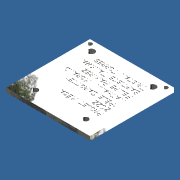
# Autodesk Inventor part: PlaqueGuideBlocLame
Saved by Autodesk Inventor 2018 (Build 220112000, 112)
## iProperties
Created: 2022-03-10
Part Number: PlaqueGuideBlocLame
Material: Aluminum 6061
Document SubType Name: Modeling
Designer: Nathann
Density: 2.7 g/cm^3
Appearance: Aluminum - Flat
Mass: 132.189 g
Surface Area: 221.993 cm^2
Volume: 48.9589 cm^3
Author: Nathann
Autodesk Inventor part; units mm, degrees
(part 1 of 3)
ref_plane "YZ Plane" through (0, 0, 0) normal (1, 0, 0) x (0, 1, 0)
ref_plane "XZ Plane" through (0, 0, 0) normal (0, 1, 0) x (-1, 0, 0)
ref_plane "XY Plane" through (0, 0, 0) normal (0, 0, 1) x (1, 0, 0)
sketch "Sketch1" plane through (0, 0, 0) normal (0, 0, 1) x (1, 0, 0)
  line L0 (0, 0) -> (-100, 0)
  line L1 (-100, 0) -> (-100, 100)
  line L2 (-100, 100) -> (0, 100)
  line L3 (0, 100) -> (0, 0)
  dimension "d0" = 100
  dimension "d1" = 100
  constraints: 8 end point, 2 parallel, 1 horizontal, 1 perpendicular
  measures "d0" distance of L2.end L0.start
  measures "d1" distance of L1.end L2.end
extrude "Extrusion1" add sketch "Sketch1" along normal blind 5
sketch "Sketch11" plane through (-80, 15, 0) normal (0, 0, -1) x (-1, 0, 0)
  circle A0 centre (0, 0) radius 3.3
  circle A1 centre (-30, 0) radius 5 projected
  circle A2 centre (-30, 0) radius 3
  circle A3 centre (-60, 0) radius 5 projected
  circle A4 centre (-60, 0) radius 3.3
  point P0 (-80, -15)
  dimension "d101" = 6.6
  dimension "d102" = 6
  dimension "d103" = 6.6
  constraints: 3 centre point, 2 coincident
  measures "d101" diameter of A0
  measures "d102" diameter of A2
  measures "d103" diameter of A4
extrude "Extrusion11" cut sketch "Sketch11" along normal through all both and the other way through all contours A0 | A4
sketch "Sketch7" plane through (0, 0, 0) normal (0, 0, -1) x (-1, 0, 0)
  line L0 (100, 25) -> (0, 25)
  line L1 (100, 56.2495) -> (100, 25)
  line L2 (100, 100) -> (0, 100)
  line L3 (0, 0) -> (100, 0) projected
  circle A0 centre (86.5, 88) radius 4
  circle A1 centre (86.5, 88) radius 1.65
  line L4 (50, 100) -> (50, 0)
  line L5 (100, 0) -> (0, 0) projected
  line L6 (0, 100) -> (0, 100)
  line L7 (0, 100) -> (0, 98.5)
  circle A2 centre (95, 95) radius 2.5
  line L8 (100, 0) -> (100, 100) projected
  line L9 (0, 0) -> (100, 0) projected
  line L10 (100, 0) -> (100, 100) projected
  line L11 (100, 100) -> (0, 100) projected
  line L12 (0, 100) -> (0, 0) projected
  circle A3 centre (13.5, 88) radius 4
  circle A4 centre (13.5, 88) radius 1.65
  circle A5 centre (5, 95) radius 2.5
  point P0 (95.4835, 97.4528)
  point P1 (95.4244, 97.4637)
  point P2 (0, 100)
  point P3 (0, 100)
  point P4 (4.5165, 97.4528)
  point P5 (4.5756, 97.4637)
  point P6 (0, 100)
  dimension "d72" = 25
  dimension "d77" = 8
  dimension "d78" = 3.3
  dimension "d88" = 5
  dimension "d111" = 5
  dimension "d112" = 8.5
  dimension "d121" = 7
  dimension "d122" = 5
  constraints: 12 end point, 8 symmetric about line, 6 centre point, 4 point on circle, 2 coincident, 2 horizontal, 2 midpoint, 3 other
  measures "d72" distance between parallel lines of L0 L3
  measures "d77" diameter of A0
  measures "d78" diameter of A1
  measures "d88" diameter of A2
  measures "d111" distance from line of L8 A2.centre
  measures "d112" horizontal distance of A2.centre A0.centre
  measures "d121" vertical distance of A0.centre A2.centre
  measures "d122" distance from line of L2 A2.centre
extrude "Extrusion13" cut sketch "Sketch7" against normal blind 10 contours A0 | A1 | A2 | A3 | A4 | A5
sketch "Sketch13" plane through (0, 0, 5) normal (0, 0, 1) x (1, 0, 0)
  line L0 (-10, 25) -> (-90, 25) construction
  line L1 (-90, 25) -> (-90, 85) construction
  line L2 (-90, 85) -> (-10, 85) construction
  line L3 (-10, 85) -> (-10, 25) construction
  line L4 (0, 0) -> (0, 100) projected
  line L5 (-100, 100) -> (-100, 0) projected
  line L6 (-100, 0) -> (0, 0) projected
  spline S0 degree 2 poles (-14.4043, 27.4336) (-14.4043, 28.1165) (-14.0606, 28.4281) knots 0 0 0 1 1 1
  spline S1 degree 2 poles (-14.0606, 28.4281) (-13.6527, 28.9735) (-12.9606, 28.9735) knots 0 0 0 1 1 1
  line L7 (-12.9606, 28.9735) -> (-11.1778, 28.9735)
  line L8 (-11.1778, 28.9735) -> (-11.1778, 31.5446)
  spline S2 degree 2 poles (-11.1778, 31.5446) (-11.1778, 31.9066) (-10.8295, 31.9066) knots 0 0 0 1 1 1
  spline S3 degree 2 poles (-10.8295, 31.9066) (-10.4766, 31.9066) (-10.4766, 31.5446) knots 0 0 0 1 1 1
  line L9 (-10.4766, 31.5446) -> (-10.4766, 25.8249)
  line L10 (-10.4766, 25.8249) -> (-12.8186, 25.8249)
  spline S4 degree 2 poles (-12.8186, 25.8249) (-13.6114, 25.8249) (-14.0285, 26.2832) knots 0 0 0 1 1 1
  spline S5 degree 2 poles (-14.0285, 26.2832) (-14.4043, 26.7095) (-14.4043, 27.4336) knots 0 0 0 1 1 1
  spline S6 degree 2 poles (-13.7031, 27.4336) (-13.7031, 26.5307) (-12.8186, 26.5307) knots 0 0 0 1 1 1
  line L11 (-12.8186, 26.5307) -> (-11.1778, 26.5307)
  line L12 (-11.1778, 26.5307) -> (-11.1778, 28.2585)
  line L13 (-11.1778, 28.2585) -> (-12.9652, 28.2585)
  spline S7 degree 2 poles (-12.9652, 28.2585) (-13.3181, 28.2585) (-13.7031, 27.814) (-13.7031, 27.4336) knots 0 0 0 1 2 2 2
  spline S8 degree 2 poles (-18.9415, 28.3089) (-18.9415, 29.0651) (-18.4694, 29.4134) knots 0 0 0 1 1 1
  spline S9 degree 2 poles (-18.4694, 29.4134) (-18.0936, 29.7205) (-17.7499, 29.7205) knots 0 0 0 1 1 1
  line L14 (-17.7499, 29.7205) -> (-17.7086, 29.7159)
  line L15 (-17.7086, 29.7159) -> (-18.8727, 31.3337)
  spline S10 degree 2 poles (-18.8727, 31.3337) (-18.9415, 31.4437) (-18.9415, 31.5446) knots 0 0 0 1 1 1
  spline S11 degree 2 poles (-18.9415, 31.5446) (-18.9415, 31.6912) (-18.7261, 31.9066) (-18.584, 31.9066) knots 0 0 0 1 2 2 2
  spline S12 degree 2 poles (-18.584, 31.9066) (-18.419, 31.9066) (-18.3778, 31.7966) knots 0 0 0 1 1 1
  line L16 (-18.3778, 31.7966) -> (-16.9295, 29.7205)
  line L17 (-16.9295, 29.7205) -> (-16.0817, 29.7205)
  line L18 (-16.0817, 29.7205) -> (-16.0817, 31.5446)
  spline S13 degree 2 poles (-16.0817, 31.5446) (-16.0817, 31.9066) (-15.7334, 31.9066) knots 0 0 0 1 1 1
  spline S14 degree 2 poles (-15.7334, 31.9066) (-15.385, 31.9066) (-15.385, 31.5446) knots 0 0 0 1 1 1
  line L19 (-15.385, 31.5446) -> (-15.385, 26.8928)
  line L20 (-15.385, 26.8928) -> (-17.4932, 26.8928)
  spline S15 degree 2 poles (-17.4932, 26.8928) (-18.0936, 26.8928) (-18.4969, 27.2503) knots 0 0 0 1 1 1
  spline S16 degree 2 poles (-18.4969, 27.2503) (-18.9415, 27.649) (-18.9415, 28.3089) knots 0 0 0 1 1 1
  spline S17 degree 2 poles (-18.2449, 28.3089) (-18.2449, 27.9652) (-17.8095, 27.5986) (-17.4932, 27.5986) knots 0 0 0 1 2 2 2
  line L21 (-17.4932, 27.5986) -> (-16.0817, 27.5986)
  line L22 (-16.0817, 27.5986) -> (-16.0817, 29.0147)
  line L23 (-16.0817, 29.0147) -> (-17.7499, 29.0147)
  spline S18 degree 2 poles (-17.7499, 29.0147) (-17.8782, 29.0147) (-18.0386, 28.8681) knots 0 0 0 1 1 1
  spline S19 degree 2 poles (-18.0386, 28.8681) (-18.2449, 28.6756) (-18.2449, 28.3089) knots 0 0 0 1 1 1
  spline S20 degree 2 poles (-23.3458, 29.3951) (-23.3458, 30.3667) (-22.8554, 31.0954) knots 0 0 0 1 1 1
  spline S21 degree 2 poles (-22.8554, 31.0954) (-22.3146, 31.8974) (-21.4667, 31.8974) knots 0 0 0 1 1 1
  spline S22 degree 2 poles (-21.4667, 31.8974) (-20.6189, 31.8974) (-20.0781, 31.0863) knots 0 0 0 1 1 1
  spline S23 degree 2 poles (-20.0781, 31.0863) (-19.5923, 30.3576) (-19.5923, 29.3951) knots 0 0 0 1 1 1
  spline S24 degree 2 poles (-19.5923, 29.3951) (-19.5923, 28.4373) (-20.0735, 27.7269) knots 0 0 0 1 1 1
  spline S25 degree 2 poles (-20.0735, 27.7269) (-20.6372, 26.9065) (-21.4667, 26.9065) knots 0 0 0 1 1 1
  spline S26 degree 2 poles (-21.4667, 26.9065) (-22.3512, 26.9065) (-22.8233, 27.6719) knots 0 0 0 1 1 1
  spline S27 degree 2 poles (-22.8233, 27.6719) (-23.3458, 28.4235) (-23.3458, 29.3951) knots 0 0 0 1 1 1
  spline S28 degree 2 poles (-22.6491, 29.3951) (-22.6491, 28.6802) (-22.3833, 28.2219) knots 0 0 0 1 1 1
  spline S29 degree 2 poles (-22.3833, 28.2219) (-22.0396, 27.6123) (-21.4667, 27.6123) knots 0 0 0 1 1 1
  spline S30 degree 2 poles (-21.4667, 27.6123) (-20.9305, 27.6123) (-20.5914, 28.1806) knots 0 0 0 1 1 1
  spline S31 degree 2 poles (-20.5914, 28.1806) (-20.2889, 28.6939) (-20.2889, 29.3951) knots 0 0 0 1 1 1
  spline S32 degree 2 poles (-20.2889, 29.3951) (-20.2889, 30.1147) (-20.4447, 30.5821) knots 0 0 0 1 1 1
  spline S33 degree 2 poles (-20.4447, 30.5821) (-20.9122, 31.1917) (-21.4667, 31.1917) knots 0 0 0 1 1 1
  spline S34 degree 2 poles (-21.4667, 31.1917) (-22.0258, 31.1917) (-22.4933, 30.5821) knots 0 0 0 1 1 1
  spline S35 degree 2 poles (-22.4933, 30.5821) (-22.6491, 30.1101) (-22.6491, 29.3951) knots 0 0 0 1 1 1
  spline S36 degree 2 poles (-27.2597, 30.1788) (-27.2597, 30.8113) (-26.8105, 31.2696) knots 0 0 0 1 1 1
  spline S37 degree 2 poles (-26.8105, 31.2696) (-26.2835, 31.9158) (-25.5227, 31.9158) knots 0 0 0 1 1 1
  spline S38 degree 2 poles (-25.5227, 31.9158) (-24.8857, 31.9158) (-24.3953, 31.3887) knots 0 0 0 1 1 1
  spline S39 degree 2 poles (-24.3953, 31.3887) (-23.9324, 30.8892) (-23.9324, 30.3484) knots 0 0 0 1 1 1
  spline S40 degree 2 poles (-23.9324, 30.3484) (-23.9324, 29.9955) (-24.2715, 29.9955) knots 0 0 0 1 1 1
  spline S41 degree 2 poles (-24.2715, 29.9955) (-24.629, 29.9955) (-24.629, 30.3667) knots 0 0 0 1 1 1
  spline S42 degree 2 poles (-24.629, 30.3667) (-24.629, 30.6554) (-25.1744, 31.2192) (-25.5273, 31.2192) knots 0 0 0 1 2 2 2
  spline S43 degree 2 poles (-25.5273, 31.2192) (-25.9764, 31.2192) (-26.2606, 30.9213) knots 0 0 0 1 1 1
  spline S44 degree 2 poles (-26.2606, 30.9213) (-26.563, 30.5592) (-26.563, 30.1788) knots 0 0 0 1 1 1
  line L24 (-26.563, 30.1788) -> (-26.563, 27.2457)
  spline S45 degree 2 poles (-26.563, 27.2457) (-26.563, 26.8836) (-26.9113, 26.8836) knots 0 0 0 1 1 1
  spline S46 degree 2 poles (-26.9113, 26.8836) (-27.2597, 26.8836) (-27.2597, 27.2457) knots 0 0 0 1 1 1
  line L25 (-27.2597, 27.2457) -> (-27.2597, 30.1788)
  line L26 (-31.224, 31.8287) -> (-28.2404, 31.8287)
  line L27 (-28.2404, 31.8287) -> (-28.2404, 26.8928)
  line L28 (-28.2404, 26.8928) -> (-31.224, 26.8928)
  spline S47 degree 2 poles (-31.224, 26.8928) (-31.5814, 26.8928) (-31.5814, 27.2365) knots 0 0 0 1 1 1
  spline S48 degree 2 poles (-31.5814, 27.2365) (-31.5814, 27.5894) (-31.224, 27.5894) knots 0 0 0 1 1 1
  line L29 (-31.224, 27.5894) -> (-28.937, 27.5894)
  line L30 (-28.937, 27.5894) -> (-28.937, 28.7489)
  line L31 (-28.937, 28.7489) -> (-31.0865, 28.7489)
  spline S49 degree 2 poles (-31.0865, 28.7489) (-31.4348, 28.7489) (-31.4348, 29.1018) knots 0 0 0 1 1 1
  spline S50 degree 2 poles (-31.4348, 29.1018) (-31.4348, 29.4547) (-31.0865, 29.4547) knots 0 0 0 1 1 1
  line L32 (-31.0865, 29.4547) -> (-28.937, 29.4547)
  line L33 (-28.937, 29.4547) -> (-28.937, 31.1229)
  line L34 (-28.937, 31.1229) -> (-31.224, 31.1229)
  spline S51 degree 2 poles (-31.224, 31.1229) (-31.5814, 31.1229) (-31.5814, 31.4758) knots 0 0 0 1 1 1
  spline S52 degree 2 poles (-31.5814, 31.4758) (-31.5814, 31.8287) (-31.224, 31.8287) knots 0 0 0 1 1 1
  line L35 (-35.8803, 27.6169) -> (-34.6979, 27.6169)
  line L36 (-34.6979, 27.6169) -> (-34.6979, 31.5446)
  spline S53 degree 2 poles (-34.6979, 31.5446) (-34.6979, 31.9158) (-34.3404, 31.9158) knots 0 0 0 1 1 1
  spline S54 degree 2 poles (-34.3404, 31.9158) (-33.9784, 31.9158) (-33.9784, 31.5446) knots 0 0 0 1 1 1
  line L37 (-33.9784, 31.5446) -> (-33.9784, 27.6169)
  line L38 (-33.9784, 27.6169) -> (-32.8005, 27.6169)
  spline S55 degree 2 poles (-32.8005, 27.6169) (-32.4385, 27.6169) (-32.4385, 27.2548) knots 0 0 0 1 1 1
  spline S56 degree 2 poles (-32.4385, 27.2548) (-32.4385, 26.8928) (-32.8005, 26.8928) knots 0 0 0 1 1 1
  line L39 (-32.8005, 26.8928) -> (-35.8803, 26.8928)
  spline S57 degree 2 poles (-35.8803, 26.8928) (-36.247, 26.8928) (-36.247, 27.2548) knots 0 0 0 1 1 1
  spline S58 degree 2 poles (-36.247, 27.2548) (-36.247, 27.6169) (-35.8803, 27.6169) knots 0 0 0 1 1 1
  spline S59 degree 2 poles (-45.3992, 31.5446) (-45.3992, 31.9066) (-45.0509, 31.9066) knots 0 0 0 1 1 1
  spline S60 degree 2 poles (-45.0509, 31.9066) (-44.698, 31.9066) (-44.698, 31.5446) knots 0 0 0 1 1 1
  line L40 (-44.698, 31.5446) -> (-44.698, 26.9386)
  line L41 (-44.698, 26.9386) -> (-43.3094, 29.1339)
  spline S61 degree 2 poles (-43.3094, 29.1339) (-43.149, 29.3676) (-42.9198, 29.3676) knots 0 0 0 1 1 1
  spline S62 degree 2 poles (-42.9198, 29.3676) (-42.6999, 29.3676) (-42.5853, 29.198) knots 0 0 0 1 1 1
  line L42 (-42.5853, 29.198) -> (-41.1691, 26.9203)
  line L43 (-41.1691, 26.9203) -> (-41.1691, 31.5446)
  spline S63 degree 2 poles (-41.1691, 31.5446) (-41.1691, 31.9066) (-40.8116, 31.9066) knots 0 0 0 1 1 1
  spline S64 degree 2 poles (-40.8116, 31.9066) (-40.4588, 31.9066) (-40.4588, 31.5446) knots 0 0 0 1 1 1
  line L44 (-40.4588, 31.5446) -> (-40.4588, 26.2237)
  spline S65 degree 2 poles (-40.4588, 26.2237) (-40.4588, 25.8433) (-40.8391, 25.8433) knots 0 0 0 1 1 1
  spline S66 degree 2 poles (-40.8391, 25.8433) (-41.1325, 25.8433) (-41.3249, 26.1137) knots 0 0 0 1 1 1
  line L45 (-41.3249, 26.1137) -> (-42.929, 28.4831)
  line L46 (-42.929, 28.4831) -> (-44.5697, 26.0862)
  spline S67 degree 2 poles (-44.5697, 26.0862) (-44.7576, 25.8066) (-45.0234, 25.8066) knots 0 0 0 1 1 1
  spline S68 degree 2 poles (-45.0234, 25.8066) (-45.3992, 25.8066) (-45.3992, 26.2191) knots 0 0 0 1 1 1
  line L47 (-45.3992, 26.2191) -> (-45.3992, 31.5446)
  line L48 (-49.744, 31.8287) -> (-46.7604, 31.8287)
  line L49 (-46.7604, 31.8287) -> (-46.7604, 26.8928)
  line L50 (-46.7604, 26.8928) -> (-49.744, 26.8928)
  spline S69 degree 2 poles (-49.744, 26.8928) (-50.1014, 26.8928) (-50.1014, 27.2365) knots 0 0 0 1 1 1
  spline S70 degree 2 poles (-50.1014, 27.2365) (-50.1014, 27.5894) (-49.744, 27.5894) knots 0 0 0 1 1 1
  line L51 (-49.744, 27.5894) -> (-47.457, 27.5894)
  line L52 (-47.457, 27.5894) -> (-47.457, 28.7489)
  line L53 (-47.457, 28.7489) -> (-49.6065, 28.7489)
  spline S71 degree 2 poles (-49.6065, 28.7489) (-49.9548, 28.7489) (-49.9548, 29.1018) knots 0 0 0 1 1 1
  spline S72 degree 2 poles (-49.9548, 29.1018) (-49.9548, 29.4547) (-49.6065, 29.4547) knots 0 0 0 1 1 1
  line L54 (-49.6065, 29.4547) -> (-47.457, 29.4547)
  line L55 (-47.457, 29.4547) -> (-47.457, 31.1229)
  line L56 (-47.457, 31.1229) -> (-49.744, 31.1229)
  spline S73 degree 2 poles (-49.744, 31.1229) (-50.1014, 31.1229) (-50.1014, 31.4758) knots 0 0 0 1 1 1
  spline S74 degree 2 poles (-50.1014, 31.4758) (-50.1014, 31.8287) (-49.744, 31.8287) knots 0 0 0 1 1 1
  line L57 (-49.5286, 25.6462) -> (-48.3782, 26.2557)
  spline S75 degree 2 poles (-48.3782, 26.2557) (-48.2866, 26.3016) (-48.2041, 26.3016) knots 0 0 0 1 1 1
  spline S76 degree 2 poles (-48.2041, 26.3016) (-48.062, 26.3016) (-47.8695, 26.0724) (-47.8695, 25.9395) knots 0 0 0 1 2 2 2
  spline S77 degree 2 poles (-47.8695, 25.9395) (-47.8695, 25.7608) (-48.0528, 25.6554) knots 0 0 0 1 1 1
  line L58 (-48.0528, 25.6554) -> (-49.194, 25.0367)
  spline S78 degree 2 poles (-49.194, 25.0367) (-49.2673, 25) (-49.3498, 25) knots 0 0 0 1 1 1
  spline S79 degree 2 poles (-49.3498, 25) (-49.4965, 25) (-49.689, 25.2292) (-49.689, 25.3712) knots 0 0 0 1 2 2 2
  spline S80 degree 2 poles (-49.689, 25.3712) (-49.689, 25.55) (-49.5286, 25.6462) knots 0 0 0 1 1 1
  spline S81 degree 2 poles (-54.5011, 31.0954) (-54.107, 31.5721) (-53.4104, 31.9158) (-52.92, 31.9158) knots 0 0 0 1 2 2 2
  spline S82 degree 2 poles (-52.92, 31.9158) (-52.1271, 31.9158) (-51.1143, 30.5088) (-51.1143, 29.3539) knots 0 0 0 1 2 2 2
  spline S83 degree 2 poles (-51.1143, 29.3539) (-51.1143, 28.0798) (-51.7192, 27.4198) knots 0 0 0 1 1 1
  spline S84 degree 2 poles (-51.7192, 27.4198) (-52.2096, 26.8836) (-52.92, 26.8836) knots 0 0 0 1 1 1
  spline S85 degree 2 poles (-52.92, 26.8836) (-53.4516, 26.8836) (-54.1253, 27.2594) (-54.3911, 27.7406) knots 0 0 0 1 2 2 2
  spline S86 degree 2 poles (-54.3911, 27.7406) (-54.4324, 27.8186) (-54.4324, 27.9056) knots 0 0 0 1 1 1
  spline S87 degree 2 poles (-54.4324, 27.9056) (-54.4324, 28.0477) (-54.2124, 28.2539) (-54.0749, 28.2539) knots 0 0 0 1 2 2 2
  spline S88 degree 2 poles (-54.0749, 28.2539) (-53.8824, 28.2539) (-53.7816, 28.0706) knots 0 0 0 1 1 1
  spline S89 degree 2 poles (-53.7816, 28.0706) (-53.5112, 27.5894) (-52.9383, 27.5894) knots 0 0 0 1 1 1
  spline S90 degree 2 poles (-52.9383, 27.5894) (-52.4983, 27.5894) (-52.205, 27.9515) knots 0 0 0 1 1 1
  spline S91 degree 2 poles (-52.205, 27.9515) (-51.8155, 28.4418) (-51.8155, 29.3539) knots 0 0 0 1 1 1
  spline S92 degree 2 poles (-51.8155, 29.3539) (-51.8155, 30.1926) (-52.4708, 31.2192) (-52.9383, 31.2192) knots 0 0 0 1 2 2 2
  spline S93 degree 2 poles (-52.9383, 31.2192) (-53.5204, 31.2192) (-53.9099, 30.8021) knots 0 0 0 1 1 1
  spline S94 degree 2 poles (-53.9099, 30.8021) (-54.0382, 30.5363) (-54.2032, 30.5363) knots 0 0 0 1 1 1
  spline S95 degree 2 poles (-54.2032, 30.5363) (-54.3407, 30.5363) (-54.5699, 30.7517) (-54.5699, 30.8983) knots 0 0 0 1 2 2 2
  spline S96 degree 2 poles (-54.5699, 30.8983) (-54.5699, 31.0267) (-54.5011, 31.0954) knots 0 0 0 1 1 1
  spline S97 degree 2 poles (-59.492, 31.4208) (-59.515, 31.4896) (-59.515, 31.5537) knots 0 0 0 1 1 1
  spline S98 degree 2 poles (-59.515, 31.5537) (-59.515, 31.705) (-59.2858, 31.8974) (-59.1483, 31.8974) knots 0 0 0 1 2 2 2
  spline S99 degree 2 poles (-59.1483, 31.8974) (-58.9146, 31.8974) (-58.8367, 31.6775) knots 0 0 0 1 1 1
  line L59 (-58.8367, 31.6775) -> (-58.5525, 30.9854)
  line L60 (-58.5525, 30.9854) -> (-56.316, 30.9854)
  line L61 (-56.316, 30.9854) -> (-56.0548, 31.6729)
  spline S100 degree 2 poles (-56.0548, 31.6729) (-55.9585, 31.8974) (-55.7248, 31.8974) knots 0 0 0 1 1 1
  spline S101 degree 2 poles (-55.7248, 31.8974) (-55.3719, 31.8974) (-55.3719, 31.5583) knots 0 0 0 1 1 1
  spline S102 degree 2 poles (-55.3719, 31.5583) (-55.3719, 31.4941) (-55.3902, 31.4391) knots 0 0 0 1 1 1
  line L62 (-55.3902, 31.4391) -> (-57.0493, 27.0624)
  spline S103 degree 2 poles (-57.0493, 27.0624) (-57.1914, 26.847) (-57.4022, 26.847) knots 0 0 0 1 1 1
  spline S104 degree 2 poles (-57.4022, 26.847) (-57.613, 26.847) (-57.7597, 27.0578) knots 0 0 0 1 1 1
  line L63 (-57.7597, 27.0578) -> (-59.492, 31.4208)
  line L64 (-58.3188, 30.2888) -> (-57.4113, 27.9011)
  line L65 (-57.4113, 27.9011) -> (-56.5314, 30.2888)
  line L66 (-56.5314, 30.2888) -> (-58.3188, 30.2888)
  line L67 (-74.0202, 31.8195) -> (-70.6563, 31.8195)
  spline S105 degree 2 poles (-70.6563, 31.8195) (-70.8029, 31.1687) (-70.9496, 30.6371) knots 0 0 0 1 1 1
  spline S106 degree 2 poles (-70.9496, 30.6371) (-71.1879, 29.8947) (-71.6095, 29.3493) knots 0 0 0 1 1 1
  spline S107 degree 2 poles (-71.6095, 29.3493) (-72.1687, 28.6298) (-73.1494, 28.0798) knots 0 0 0 1 1 1
  spline S108 degree 2 poles (-73.1494, 28.0798) (-73.6902, 27.7773) (-73.6902, 27.264) knots 0 0 0 1 1 1
  spline S109 degree 2 poles (-73.6902, 27.264) (-73.6902, 26.9478) (-73.4473, 26.7049) knots 0 0 0 1 1 1
  spline S110 degree 2 poles (-73.4473, 26.7049) (-73.2182, 26.4895) (-72.8057, 26.4895) knots 0 0 0 1 1 1
  spline S111 degree 2 poles (-72.8057, 26.4895) (-72.3428, 26.4895) (-72.0678, 26.6316) knots 0 0 0 1 1 1
  spline S112 degree 2 poles (-72.0678, 26.6316) (-71.7974, 26.7874) (-71.6279, 27.1219) knots 0 0 0 1 1 1
  spline S113 degree 2 poles (-71.6279, 27.1219) (-71.527, 27.4427) (-71.3116, 27.4427) knots 0 0 0 1 1 1
  spline S114 degree 2 poles (-71.3116, 27.4427) (-70.9588, 27.4427) (-70.9588, 27.099) knots 0 0 0 1 1 1
  spline S115 degree 2 poles (-70.9588, 27.099) (-70.9588, 27.0303) (-70.9817, 27.0028) knots 0 0 0 1 1 1
  spline S116 degree 2 poles (-70.9817, 27.0028) (-71.4766, 25.7745) (-72.7736, 25.7745) knots 0 0 0 1 1 1
  spline S117 degree 2 poles (-72.7736, 25.7745) (-73.539, 25.7745) (-74.0019, 26.2099) knots 0 0 0 1 1 1
  spline S118 degree 2 poles (-74.0019, 26.2099) (-74.4373, 26.6178) (-74.4373, 27.2182) knots 0 0 0 1 1 1
  spline S119 degree 2 poles (-74.4373, 27.2182) (-74.4373, 28.1531) (-73.4886, 28.6985) knots 0 0 0 1 1 1
  spline S120 degree 2 poles (-73.4886, 28.6985) (-72.4528, 29.2851) (-71.9441, 30.0826) knots 0 0 0 1 1 1
  spline S121 degree 2 poles (-71.9441, 30.0826) (-71.7654, 30.4171) (-71.55, 31.1137) knots 0 0 0 1 1 1
  line L68 (-71.55, 31.1137) -> (-74.0202, 31.1137)
  spline S122 degree 2 poles (-74.0202, 31.1137) (-74.3777, 31.1137) (-74.3777, 31.4666) knots 0 0 0 1 1 1
  spline S123 degree 2 poles (-74.3777, 31.4666) (-74.3777, 31.8195) (-74.0202, 31.8195) knots 0 0 0 1 1 1
  spline S124 degree 2 poles (-79.2953, 28.8864) (-79.2953, 30.1101) (-78.8186, 30.9763) knots 0 0 0 1 1 1
  spline S125 degree 2 poles (-78.8186, 30.9763) (-78.287, 31.9387) (-77.4254, 31.9387) knots 0 0 0 1 1 1
  spline S126 degree 2 poles (-77.4254, 31.9387) (-76.5638, 31.9387) (-76.0276, 30.9763) knots 0 0 0 1 1 1
  spline S127 degree 2 poles (-76.0276, 30.9763) (-75.5555, 30.1055) (-75.5555, 28.8864) knots 0 0 0 1 1 1
  spline S128 degree 2 poles (-75.5555, 28.8864) (-75.5555, 27.6765) (-76.0367, 26.8011) knots 0 0 0 1 1 1
  spline S129 degree 2 poles (-76.0367, 26.8011) (-76.573, 25.8249) (-77.4254, 25.8249) knots 0 0 0 1 1 1
  spline S130 degree 2 poles (-77.4254, 25.8249) (-78.287, 25.8249) (-78.8186, 26.8011) knots 0 0 0 1 1 1
  spline S131 degree 2 poles (-78.8186, 26.8011) (-79.2953, 27.6719) (-79.2953, 28.8864) knots 0 0 0 1 1 1
  spline S132 degree 2 poles (-78.5986, 28.8772) (-78.5986, 27.9285) (-78.2733, 27.1219) knots 0 0 0 1 1 1
  spline S133 degree 2 poles (-78.2733, 27.1219) (-77.9479, 26.5399) (-77.4208, 26.5399) knots 0 0 0 1 1 1
  spline S134 degree 2 poles (-77.4208, 26.5399) (-76.9029, 26.5399) (-76.5821, 27.1632) knots 0 0 0 1 1 1
  spline S135 degree 2 poles (-76.5821, 27.1632) (-76.2567, 27.9331) (-76.2567, 28.8864) knots 0 0 0 1 1 1
  spline S136 degree 2 poles (-76.2567, 28.8864) (-76.2567, 29.8443) (-76.5821, 30.6096) knots 0 0 0 1 1 1
  spline S137 degree 2 poles (-76.5821, 30.6096) (-76.9029, 31.2329) (-77.4208, 31.2329) knots 0 0 0 1 1 1
  spline S138 degree 2 poles (-77.4208, 31.2329) (-77.9433, 31.2329) (-78.2733, 30.605) knots 0 0 0 1 1 1
  spline S139 degree 2 poles (-78.2733, 30.605) (-78.5986, 29.8305) (-78.5986, 28.8772) knots 0 0 0 1 1 1
  line L69 (-83.6079, 31.8195) -> (-80.244, 31.8195)
  spline S140 degree 2 poles (-80.244, 31.8195) (-80.3906, 31.1687) (-80.5373, 30.6371) knots 0 0 0 1 1 1
  spline S141 degree 2 poles (-80.5373, 30.6371) (-80.7756, 29.8947) (-81.1972, 29.3493) knots 0 0 0 1 1 1
  spline S142 degree 2 poles (-81.1972, 29.3493) (-81.7564, 28.6298) (-82.7371, 28.0798) knots 0 0 0 1 1 1
  spline S143 degree 2 poles (-82.7371, 28.0798) (-83.2779, 27.7773) (-83.2779, 27.264) knots 0 0 0 1 1 1
  spline S144 degree 2 poles (-83.2779, 27.264) (-83.2779, 26.9478) (-83.035, 26.7049) knots 0 0 0 1 1 1
  spline S145 degree 2 poles (-83.035, 26.7049) (-82.8059, 26.4895) (-82.3934, 26.4895) knots 0 0 0 1 1 1
  spline S146 degree 2 poles (-82.3934, 26.4895) (-81.9305, 26.4895) (-81.6555, 26.6316) knots 0 0 0 1 1 1
  spline S147 degree 2 poles (-81.6555, 26.6316) (-81.3851, 26.7874) (-81.2156, 27.1219) knots 0 0 0 1 1 1
  spline S148 degree 2 poles (-81.2156, 27.1219) (-81.1147, 27.4427) (-80.8993, 27.4427) knots 0 0 0 1 1 1
  spline S149 degree 2 poles (-80.8993, 27.4427) (-80.5464, 27.4427) (-80.5464, 27.099) knots 0 0 0 1 1 1
  spline S150 degree 2 poles (-80.5464, 27.099) (-80.5464, 27.0303) (-80.5693, 27.0028) knots 0 0 0 1 1 1
  spline S151 degree 2 poles (-80.5693, 27.0028) (-81.0643, 25.7745) (-82.3613, 25.7745) knots 0 0 0 1 1 1
  spline S152 degree 2 poles (-82.3613, 25.7745) (-83.1267, 25.7745) (-83.5896, 26.2099) knots 0 0 0 1 1 1
  spline S153 degree 2 poles (-83.5896, 26.2099) (-84.0249, 26.6178) (-84.0249, 27.2182) knots 0 0 0 1 1 1
  spline S154 degree 2 poles (-84.0249, 27.2182) (-84.0249, 28.1531) (-83.0763, 28.6985) knots 0 0 0 1 1 1
  spline S155 degree 2 poles (-83.0763, 28.6985) (-82.0405, 29.2851) (-81.5318, 30.0826) knots 0 0 0 1 1 1
  spline S156 degree 2 poles (-81.5318, 30.0826) (-81.353, 30.4171) (-81.1376, 31.1137) knots 0 0 0 1 1 1
  line L70 (-81.1376, 31.1137) -> (-83.6079, 31.1137)
  spline S157 degree 2 poles (-83.6079, 31.1137) (-83.9654, 31.1137) (-83.9654, 31.4666) knots 0 0 0 1 1 1
  spline S158 degree 2 poles (-83.9654, 31.4666) (-83.9654, 31.8195) (-83.6079, 31.8195) knots 0 0 0 1 1 1
  line L71 (-88.4017, 31.8195) -> (-85.0378, 31.8195)
  spline S159 degree 2 poles (-85.0378, 31.8195) (-85.1844, 31.1687) (-85.3311, 30.6371) knots 0 0 0 1 1 1
  spline S160 degree 2 poles (-85.3311, 30.6371) (-85.5694, 29.8947) (-85.9911, 29.3493) knots 0 0 0 1 1 1
  spline S161 degree 2 poles (-85.9911, 29.3493) (-86.5502, 28.6298) (-87.531, 28.0798) knots 0 0 0 1 1 1
  spline S162 degree 2 poles (-87.531, 28.0798) (-88.0718, 27.7773) (-88.0718, 27.264) knots 0 0 0 1 1 1
  spline S163 degree 2 poles (-88.0718, 27.264) (-88.0718, 26.9478) (-87.8289, 26.7049) knots 0 0 0 1 1 1
  spline S164 degree 2 poles (-87.8289, 26.7049) (-87.5997, 26.4895) (-87.1872, 26.4895) knots 0 0 0 1 1 1
  spline S165 degree 2 poles (-87.1872, 26.4895) (-86.7243, 26.4895) (-86.4494, 26.6316) knots 0 0 0 1 1 1
  spline S166 degree 2 poles (-86.4494, 26.6316) (-86.179, 26.7874) (-86.0094, 27.1219) knots 0 0 0 1 1 1
  spline S167 degree 2 poles (-86.0094, 27.1219) (-85.9086, 27.4427) (-85.6932, 27.4427) knots 0 0 0 1 1 1
  spline S168 degree 2 poles (-85.6932, 27.4427) (-85.3403, 27.4427) (-85.3403, 27.099) knots 0 0 0 1 1 1
  spline S169 degree 2 poles (-85.3403, 27.099) (-85.3403, 27.0303) (-85.3632, 27.0028) knots 0 0 0 1 1 1
  spline S170 degree 2 poles (-85.3632, 27.0028) (-85.8582, 25.7745) (-87.1551, 25.7745) knots 0 0 0 1 1 1
  spline S171 degree 2 poles (-87.1551, 25.7745) (-87.9205, 25.7745) (-88.3834, 26.2099) knots 0 0 0 1 1 1
  spline S172 degree 2 poles (-88.3834, 26.2099) (-88.8188, 26.6178) (-88.8188, 27.2182) knots 0 0 0 1 1 1
  spline S173 degree 2 poles (-88.8188, 27.2182) (-88.8188, 28.1531) (-87.8701, 28.6985) knots 0 0 0 1 1 1
  spline S174 degree 2 poles (-87.8701, 28.6985) (-86.8343, 29.2851) (-86.3256, 30.0826) knots 0 0 0 1 1 1
  spline S175 degree 2 poles (-86.3256, 30.0826) (-86.1469, 30.4171) (-85.9315, 31.1137) knots 0 0 0 1 1 1
  line L72 (-85.9315, 31.1137) -> (-88.4017, 31.1137)
  spline S176 degree 2 poles (-88.4017, 31.1137) (-88.7592, 31.1137) (-88.7592, 31.4666) knots 0 0 0 1 1 1
  spline S177 degree 2 poles (-88.7592, 31.4666) (-88.7592, 31.8195) (-88.4017, 31.8195) knots 0 0 0 1 1 1
  spline S178 degree 2 poles (-11.2649, 36.306) (-11.2649, 36.6406) (-10.9074, 36.6406) knots 0 0 0 1 1 1
  spline S179 degree 2 poles (-10.9074, 36.6406) (-10.5545, 36.6406) (-10.5545, 36.306) knots 0 0 0 1 1 1
  line L73 (-10.5545, 36.306) -> (-10.5545, 34.9082)
  spline S180 degree 2 poles (-10.5545, 34.9082) (-10.5545, 34.5737) (-10.9074, 34.5737) knots 0 0 0 1 1 1
  spline S181 degree 2 poles (-10.9074, 34.5737) (-11.2649, 34.5737) (-11.2649, 34.9082) knots 0 0 0 1 1 1
  line L74 (-11.2649, 34.9082) -> (-11.2649, 36.306)
  spline S182 degree 2 poles (-12.3603, 36.306) (-12.3603, 36.6406) (-12.0119, 36.6406) knots 0 0 0 1 1 1
  spline S183 degree 2 poles (-12.0119, 36.6406) (-11.6591, 36.6406) (-11.6591, 36.306) knots 0 0 0 1 1 1
  line L75 (-11.6591, 36.306) -> (-11.6591, 34.9082)
  spline S184 degree 2 poles (-11.6591, 34.9082) (-11.6591, 34.5737) (-12.0119, 34.5737) knots 0 0 0 1 1 1
  spline S185 degree 2 poles (-12.0119, 34.5737) (-12.3603, 34.5737) (-12.3603, 34.9082) knots 0 0 0 1 1 1
  line L76 (-12.3603, 34.9082) -> (-12.3603, 36.306)
  spline S186 degree 2 poles (-17.2412, 36.1823) (-17.2412, 36.8652) (-16.8974, 37.1768) knots 0 0 0 1 1 1
  spline S187 degree 2 poles (-16.8974, 37.1768) (-16.4896, 37.7222) (-15.7975, 37.7222) knots 0 0 0 1 1 1
  line L77 (-15.7975, 37.7222) -> (-14.0147, 37.7222)
  line L78 (-14.0147, 37.7222) -> (-14.0147, 40.2933)
  spline S188 degree 2 poles (-14.0147, 40.2933) (-14.0147, 40.6553) (-13.6664, 40.6553) knots 0 0 0 1 1 1
  spline S189 degree 2 poles (-13.6664, 40.6553) (-13.3135, 40.6553) (-13.3135, 40.2933) knots 0 0 0 1 1 1
  line L79 (-13.3135, 40.2933) -> (-13.3135, 34.5737)
  line L80 (-13.3135, 34.5737) -> (-15.6554, 34.5737)
  spline S190 degree 2 poles (-15.6554, 34.5737) (-16.4483, 34.5737) (-16.8654, 35.032) knots 0 0 0 1 1 1
  spline S191 degree 2 poles (-16.8654, 35.032) (-17.2412, 35.4582) (-17.2412, 36.1823) knots 0 0 0 1 1 1
  spline S192 degree 2 poles (-16.54, 36.1823) (-16.54, 35.2794) (-15.6554, 35.2794) knots 0 0 0 1 1 1
  line L81 (-15.6554, 35.2794) -> (-14.0147, 35.2794)
  line L82 (-14.0147, 35.2794) -> (-14.0147, 37.0072)
  line L83 (-14.0147, 37.0072) -> (-15.8021, 37.0072)
  spline S193 degree 2 poles (-15.8021, 37.0072) (-16.155, 37.0072) (-16.54, 36.5627) (-16.54, 36.1823) knots 0 0 0 1 2 2 2
  line L84 (-21.2101, 40.5774) -> (-18.2265, 40.5774)
  line L85 (-18.2265, 40.5774) -> (-18.2265, 35.6415)
  line L86 (-18.2265, 35.6415) -> (-21.2101, 35.6415)
  spline S194 degree 2 poles (-21.2101, 35.6415) (-21.5675, 35.6415) (-21.5675, 35.9852) knots 0 0 0 1 1 1
  spline S195 degree 2 poles (-21.5675, 35.9852) (-21.5675, 36.3381) (-21.2101, 36.3381) knots 0 0 0 1 1 1
  line L87 (-21.2101, 36.3381) -> (-18.9231, 36.3381)
  line L88 (-18.9231, 36.3381) -> (-18.9231, 37.4976)
  line L89 (-18.9231, 37.4976) -> (-21.0726, 37.4976)
  spline S196 degree 2 poles (-21.0726, 37.4976) (-21.4209, 37.4976) (-21.4209, 37.8505) knots 0 0 0 1 1 1
  spline S197 degree 2 poles (-21.4209, 37.8505) (-21.4209, 38.2034) (-21.0726, 38.2034) knots 0 0 0 1 1 1
  line L90 (-21.0726, 38.2034) -> (-18.9231, 38.2034)
  line L91 (-18.9231, 38.2034) -> (-18.9231, 39.8716)
  line L92 (-18.9231, 39.8716) -> (-21.2101, 39.8716)
  spline S198 degree 2 poles (-21.2101, 39.8716) (-21.5675, 39.8716) (-21.5675, 40.2245) knots 0 0 0 1 1 1
  spline S199 degree 2 poles (-21.5675, 40.2245) (-21.5675, 40.5774) (-21.2101, 40.5774) knots 0 0 0 1 1 1
  spline S200 degree 2 poles (-20.101, 34.4133) (-20.2889, 34.5187) (-20.2889, 34.6974) knots 0 0 0 1 1 1
  spline S201 degree 2 poles (-20.2889, 34.6974) (-20.2889, 34.8303) (-20.0964, 35.0595) (-19.9497, 35.0595) knots 0 0 0 1 2 2 2
  spline S202 degree 2 poles (-19.9497, 35.0595) (-19.8627, 35.0595) (-19.8122, 35.0274) knots 0 0 0 1 1 1
  line L93 (-19.8122, 35.0274) -> (-18.6527, 34.4133)
  spline S203 degree 2 poles (-18.6527, 34.4133) (-18.4694, 34.3078) (-18.4694, 34.1291) knots 0 0 0 1 1 1
  spline S204 degree 2 poles (-18.4694, 34.1291) (-18.4694, 33.9824) (-18.6619, 33.7579) (-18.804, 33.7579) knots 0 0 0 1 2 2 2
  spline S205 degree 2 poles (-18.804, 33.7579) (-18.8865, 33.7579) (-18.9598, 33.7945) knots 0 0 0 1 1 1
  line L94 (-18.9598, 33.7945) -> (-20.101, 34.4133)
  line L95 (-25.5364, 40.5774) -> (-22.5529, 40.5774)
  line L96 (-22.5529, 40.5774) -> (-22.5529, 35.9944)
  spline S206 degree 2 poles (-22.5529, 35.9944) (-22.5529, 35.6323) (-22.9012, 35.6323) knots 0 0 0 1 1 1
  spline S207 degree 2 poles (-22.9012, 35.6323) (-23.2495, 35.6323) (-23.2495, 35.9944) knots 0 0 0 1 1 1
  line L97 (-23.2495, 35.9944) -> (-23.2495, 39.8716)
  line L98 (-23.2495, 39.8716) -> (-25.5364, 39.8716)
  spline S208 degree 2 poles (-25.5364, 39.8716) (-25.8939, 39.8716) (-25.8939, 40.2245) knots 0 0 0 1 1 1
  spline S209 degree 2 poles (-25.8939, 40.2245) (-25.8939, 40.5774) (-25.5364, 40.5774) knots 0 0 0 1 1 1
  line L99 (-29.5282, 40.5774) -> (-26.5447, 40.5774)
  line L100 (-26.5447, 40.5774) -> (-26.5447, 35.6415)
  line L101 (-26.5447, 35.6415) -> (-29.5282, 35.6415)
  spline S210 degree 2 poles (-29.5282, 35.6415) (-29.8857, 35.6415) (-29.8857, 35.9852) knots 0 0 0 1 1 1
  spline S211 degree 2 poles (-29.8857, 35.9852) (-29.8857, 36.3381) (-29.5282, 36.3381) knots 0 0 0 1 1 1
  line L102 (-29.5282, 36.3381) -> (-27.2413, 36.3381)
  line L103 (-27.2413, 36.3381) -> (-27.2413, 37.4976)
  line L104 (-27.2413, 37.4976) -> (-29.3908, 37.4976)
  spline S212 degree 2 poles (-29.3908, 37.4976) (-29.7391, 37.4976) (-29.7391, 37.8505) knots 0 0 0 1 1 1
  spline S213 degree 2 poles (-29.7391, 37.8505) (-29.7391, 38.2034) (-29.3908, 38.2034) knots 0 0 0 1 1 1
  line L105 (-29.3908, 38.2034) -> (-27.2413, 38.2034)
  line L106 (-27.2413, 38.2034) -> (-27.2413, 39.8716)
  line L107 (-27.2413, 39.8716) -> (-29.5282, 39.8716)
  spline S214 degree 2 poles (-29.5282, 39.8716) (-29.8857, 39.8716) (-29.8857, 40.2245) knots 0 0 0 1 1 1
  spline S215 degree 2 poles (-29.8857, 40.2245) (-29.8857, 40.5774) (-29.5282, 40.5774) knots 0 0 0 1 1 1
  spline S216 degree 2 poles (-38.4697, 39.7204) (-38.0206, 40.2658) (-37.6081, 40.4628) knots 0 0 0 1 1 1
  spline S217 degree 2 poles (-37.6081, 40.4628) (-37.1636, 40.6874) (-36.5632, 40.6874) knots 0 0 0 1 1 1
  spline S218 degree 2 poles (-36.5632, 40.6874) (-35.5458, 40.6874) (-34.2304, 38.9642) (-34.2304, 37.548) knots 0 0 0 1 2 2 2
  spline S219 degree 2 poles (-34.2304, 37.548) (-34.2304, 36.0036) (-35.1195, 35.1603) knots 0 0 0 1 1 1
  spline S220 degree 2 poles (-35.1195, 35.1603) (-35.5778, 34.5232) (-36.4349, 34.5232) knots 0 0 0 1 1 1
  spline S221 degree 2 poles (-36.4349, 34.5232) (-37.1086, 34.5232) (-37.5394, 34.7478) knots 0 0 0 1 1 1
  spline S222 degree 2 poles (-37.5394, 34.7478) (-37.9152, 34.9311) (-38.2268, 35.4719) knots 0 0 0 1 1 1
  spline S223 degree 2 poles (-38.2268, 35.4719) (-38.2864, 35.5682) (-38.2864, 35.6598) knots 0 0 0 1 1 1
  spline S224 degree 2 poles (-38.2864, 35.6598) (-38.2864, 35.7973) (-38.071, 36.0036) (-37.9198, 36.0036) knots 0 0 0 1 2 2 2
  spline S225 degree 2 poles (-37.9198, 36.0036) (-37.7319, 36.0036) (-37.6173, 35.8065) knots 0 0 0 1 1 1
  spline S226 degree 2 poles (-37.6173, 35.8065) (-37.4294, 35.4857) (-37.1773, 35.3574) knots 0 0 0 1 1 1
  spline S227 degree 2 poles (-37.1773, 35.3574) (-36.8932, 35.2382) (-36.4303, 35.2382) knots 0 0 0 1 1 1
  spline S228 degree 2 poles (-36.4303, 35.2382) (-35.8391, 35.2382) (-35.4358, 35.7377) knots 0 0 0 1 1 1
  spline S229 degree 2 poles (-35.4358, 35.7377) (-34.9316, 36.3565) (-34.9316, 37.548) knots 0 0 0 1 1 1
  spline S230 degree 2 poles (-34.9316, 37.548) (-34.9316, 38.6342) (-35.8757, 39.9816) (-36.5769, 39.9816) knots 0 0 0 1 2 2 2
  spline S231 degree 2 poles (-36.5769, 39.9816) (-37.3515, 39.9816) (-37.9289, 39.2758) knots 0 0 0 1 1 1
  spline S232 degree 2 poles (-37.9289, 39.2758) (-38.0343, 39.1475) (-38.1856, 39.1475) knots 0 0 0 1 1 1
  spline S233 degree 2 poles (-38.1856, 39.1475) (-38.3276, 39.1475) (-38.5431, 39.3629) (-38.5431, 39.5004) knots 0 0 0 1 2 2 2
  spline S234 degree 2 poles (-38.5431, 39.5004) (-38.5431, 39.6241) (-38.4697, 39.7204) knots 0 0 0 1 1 1
  spline S235 degree 2 poles (-43.786, 40.1695) (-43.8089, 40.2383) (-43.8089, 40.3024) knots 0 0 0 1 1 1
  spline S236 degree 2 poles (-43.8089, 40.3024) (-43.8089, 40.4537) (-43.5798, 40.6462) (-43.4423, 40.6462) knots 0 0 0 1 2 2 2
  spline S237 degree 2 poles (-43.4423, 40.6462) (-43.2086, 40.6462) (-43.1307, 40.4262) knots 0 0 0 1 1 1
  line L108 (-43.1307, 40.4262) -> (-42.8465, 39.7341)
  line L109 (-42.8465, 39.7341) -> (-40.61, 39.7341)
  line L110 (-40.61, 39.7341) -> (-40.3488, 40.4216)
  spline S238 degree 2 poles (-40.3488, 40.4216) (-40.2525, 40.6462) (-40.0188, 40.6462) knots 0 0 0 1 1 1
  spline S239 degree 2 poles (-40.0188, 40.6462) (-39.6659, 40.6462) (-39.6659, 40.307) knots 0 0 0 1 1 1
  spline S240 degree 2 poles (-39.6659, 40.307) (-39.6659, 40.2429) (-39.6842, 40.1879) knots 0 0 0 1 1 1
  line L111 (-39.6842, 40.1879) -> (-41.3433, 35.8111)
  spline S241 degree 2 poles (-41.3433, 35.8111) (-41.4854, 35.5957) (-41.6962, 35.5957) knots 0 0 0 1 1 1
  spline S242 degree 2 poles (-41.6962, 35.5957) (-41.907, 35.5957) (-42.0536, 35.8065) knots 0 0 0 1 1 1
  line L112 (-42.0536, 35.8065) -> (-43.786, 40.1695)
  line L113 (-42.6128, 39.0375) -> (-41.7053, 36.6498)
  line L114 (-41.7053, 36.6498) -> (-40.8254, 39.0375)
  line L115 (-40.8254, 39.0375) -> (-42.6128, 39.0375)
  spline S243 degree 2 poles (-48.3324, 37.0577) (-48.3324, 37.8139) (-47.8603, 38.1622) knots 0 0 0 1 1 1
  spline S244 degree 2 poles (-47.8603, 38.1622) (-47.4845, 38.4692) (-47.1408, 38.4692) knots 0 0 0 1 1 1
  line L116 (-47.1408, 38.4692) -> (-47.0996, 38.4646)
  line L117 (-47.0996, 38.4646) -> (-48.2636, 40.0824)
  spline S245 degree 2 poles (-48.2636, 40.0824) (-48.3324, 40.1924) (-48.3324, 40.2933) knots 0 0 0 1 1 1
  spline S246 degree 2 poles (-48.3324, 40.2933) (-48.3324, 40.4399) (-48.117, 40.6553) (-47.9749, 40.6553) knots 0 0 0 1 2 2 2
  spline S247 degree 2 poles (-47.9749, 40.6553) (-47.8099, 40.6553) (-47.7687, 40.5453) knots 0 0 0 1 1 1
  line L118 (-47.7687, 40.5453) -> (-46.3204, 38.4692)
  line L119 (-46.3204, 38.4692) -> (-45.4726, 38.4692)
  line L120 (-45.4726, 38.4692) -> (-45.4726, 40.2933)
  spline S248 degree 2 poles (-45.4726, 40.2933) (-45.4726, 40.6553) (-45.1243, 40.6553) knots 0 0 0 1 1 1
  spline S249 degree 2 poles (-45.1243, 40.6553) (-44.776, 40.6553) (-44.776, 40.2933) knots 0 0 0 1 1 1
  line L121 (-44.776, 40.2933) -> (-44.776, 35.6415)
  line L122 (-44.776, 35.6415) -> (-46.8841, 35.6415)
  spline S250 degree 2 poles (-46.8841, 35.6415) (-47.4845, 35.6415) (-47.8878, 35.999) knots 0 0 0 1 1 1
  spline S251 degree 2 poles (-47.8878, 35.999) (-48.3324, 36.3977) (-48.3324, 37.0577) knots 0 0 0 1 1 1
  spline S252 degree 2 poles (-47.6358, 37.0577) (-47.6358, 36.7139) (-47.2004, 36.3473) (-46.8841, 36.3473) knots 0 0 0 1 2 2 2
  line L123 (-46.8841, 36.3473) -> (-45.4726, 36.3473)
  line L124 (-45.4726, 36.3473) -> (-45.4726, 37.7634)
  line L125 (-45.4726, 37.7634) -> (-47.1408, 37.7634)
  spline S253 degree 2 poles (-47.1408, 37.7634) (-47.2691, 37.7634) (-47.4295, 37.6168) knots 0 0 0 1 1 1
  spline S254 degree 2 poles (-47.4295, 37.6168) (-47.6358, 37.4243) (-47.6358, 37.0577) knots 0 0 0 1 1 1
  spline S255 degree 2 poles (-52.7367, 38.1438) (-52.7367, 39.1154) (-52.2463, 39.8441) knots 0 0 0 1 1 1
  spline S256 degree 2 poles (-52.2463, 39.8441) (-51.7055, 40.6462) (-50.8576, 40.6462) knots 0 0 0 1 1 1
  spline S257 degree 2 poles (-50.8576, 40.6462) (-50.0098, 40.6462) (-49.469, 39.835) knots 0 0 0 1 1 1
  spline S258 degree 2 poles (-49.469, 39.835) (-48.9832, 39.1063) (-48.9832, 38.1438) knots 0 0 0 1 1 1
  spline S259 degree 2 poles (-48.9832, 38.1438) (-48.9832, 37.186) (-49.4644, 36.4756) knots 0 0 0 1 1 1
  spline S260 degree 2 poles (-49.4644, 36.4756) (-50.0281, 35.6553) (-50.8576, 35.6553) knots 0 0 0 1 1 1
  spline S261 degree 2 poles (-50.8576, 35.6553) (-51.7421, 35.6553) (-52.2142, 36.4206) knots 0 0 0 1 1 1
  spline S262 degree 2 poles (-52.2142, 36.4206) (-52.7367, 37.1722) (-52.7367, 38.1438) knots 0 0 0 1 1 1
  spline S263 degree 2 poles (-52.04, 38.1438) (-52.04, 37.4289) (-51.7742, 36.9706) knots 0 0 0 1 1 1
  spline S264 degree 2 poles (-51.7742, 36.9706) (-51.4305, 36.361) (-50.8576, 36.361) knots 0 0 0 1 1 1
  spline S265 degree 2 poles (-50.8576, 36.361) (-50.3214, 36.361) (-49.9823, 36.9293) knots 0 0 0 1 1 1
  spline S266 degree 2 poles (-49.9823, 36.9293) (-49.6798, 37.4426) (-49.6798, 38.1438) knots 0 0 0 1 1 1
  spline S267 degree 2 poles (-49.6798, 38.1438) (-49.6798, 38.8634) (-49.8356, 39.3308) knots 0 0 0 1 1 1
  spline S268 degree 2 poles (-49.8356, 39.3308) (-50.3031, 39.9404) (-50.8576, 39.9404) knots 0 0 0 1 1 1
  spline S269 degree 2 poles (-50.8576, 39.9404) (-51.4168, 39.9404) (-51.8842, 39.3308) knots 0 0 0 1 1 1
  spline S270 degree 2 poles (-51.8842, 39.3308) (-52.04, 38.8588) (-52.04, 38.1438) knots 0 0 0 1 1 1
  line L126 (-56.9072, 36.3656) -> (-55.7248, 36.3656)
  line L127 (-55.7248, 36.3656) -> (-55.7248, 40.2933)
  spline S271 degree 2 poles (-55.7248, 40.2933) (-55.7248, 40.6645) (-55.3673, 40.6645) knots 0 0 0 1 1 1
  spline S272 degree 2 poles (-55.3673, 40.6645) (-55.0053, 40.6645) (-55.0053, 40.2933) knots 0 0 0 1 1 1
  line L128 (-55.0053, 40.2933) -> (-55.0053, 36.3656)
  line L129 (-55.0053, 36.3656) -> (-53.8274, 36.3656)
  spline S273 degree 2 poles (-53.8274, 36.3656) (-53.4654, 36.3656) (-53.4654, 36.0036) knots 0 0 0 1 1 1
  spline S274 degree 2 poles (-53.4654, 36.0036) (-53.4654, 35.6415) (-53.8274, 35.6415) knots 0 0 0 1 1 1
  line L130 (-53.8274, 35.6415) -> (-56.9072, 35.6415)
  spline S275 degree 2 poles (-56.9072, 35.6415) (-57.2739, 35.6415) (-57.2739, 36.0036) knots 0 0 0 1 1 1
  spline S276 degree 2 poles (-57.2739, 36.0036) (-57.2739, 36.3656) (-56.9072, 36.3656) knots 0 0 0 1 1 1
  line L131 (-61.394, 36.3656) -> (-60.2116, 36.3656)
  line L132 (-60.2116, 36.3656) -> (-60.2116, 40.2933)
  spline S277 degree 2 poles (-60.2116, 40.2933) (-60.2116, 40.6645) (-59.8541, 40.6645) knots 0 0 0 1 1 1
  spline S278 degree 2 poles (-59.8541, 40.6645) (-59.492, 40.6645) (-59.492, 40.2933) knots 0 0 0 1 1 1
  line L133 (-59.492, 40.2933) -> (-59.492, 36.3656)
  line L134 (-59.492, 36.3656) -> (-58.3142, 36.3656)
  spline S279 degree 2 poles (-58.3142, 36.3656) (-57.9521, 36.3656) (-57.9521, 36.0036) knots 0 0 0 1 1 1
  spline S280 degree 2 poles (-57.9521, 36.0036) (-57.9521, 35.6415) (-58.3142, 35.6415) knots 0 0 0 1 1 1
  line L135 (-58.3142, 35.6415) -> (-61.394, 35.6415)
  spline S281 degree 2 poles (-61.394, 35.6415) (-61.7606, 35.6415) (-61.7606, 36.0036) knots 0 0 0 1 1 1
  spline S282 degree 2 poles (-61.7606, 36.0036) (-61.7606, 36.3656) (-61.394, 36.3656) knots 0 0 0 1 1 1
  line L136 (-65.5554, 40.5774) -> (-62.5718, 40.5774)
  line L137 (-62.5718, 40.5774) -> (-62.5718, 35.6415)
  line L138 (-62.5718, 35.6415) -> (-65.5554, 35.6415)
  spline S283 degree 2 poles (-65.5554, 35.6415) (-65.9128, 35.6415) (-65.9128, 35.9852) knots 0 0 0 1 1 1
  spline S284 degree 2 poles (-65.9128, 35.9852) (-65.9128, 36.3381) (-65.5554, 36.3381) knots 0 0 0 1 1 1
  line L139 (-65.5554, 36.3381) -> (-63.2684, 36.3381)
  line L140 (-63.2684, 36.3381) -> (-63.2684, 37.4976)
  line L141 (-63.2684, 37.4976) -> (-65.4179, 37.4976)
  spline S285 degree 2 poles (-65.4179, 37.4976) (-65.7662, 37.4976) (-65.7662, 37.8505) knots 0 0 0 1 1 1
  spline S286 degree 2 poles (-65.7662, 37.8505) (-65.7662, 38.2034) (-65.4179, 38.2034) knots 0 0 0 1 1 1
  line L142 (-65.4179, 38.2034) -> (-63.2684, 38.2034)
  line L143 (-63.2684, 38.2034) -> (-63.2684, 39.8716)
  line L144 (-63.2684, 39.8716) -> (-65.5554, 39.8716)
  spline S287 degree 2 poles (-65.5554, 39.8716) (-65.9128, 39.8716) (-65.9128, 40.2245) knots 0 0 0 1 1 1
  spline S288 degree 2 poles (-65.9128, 40.2245) (-65.9128, 40.5774) (-65.5554, 40.5774) knots 0 0 0 1 1 1
  spline S289 degree 2 poles (-67.6498, 36.306) (-67.6498, 36.6406) (-67.2923, 36.6406) knots 0 0 0 1 1 1
  spline S290 degree 2 poles (-67.2923, 36.6406) (-66.9394, 36.6406) (-66.9394, 36.306) knots 0 0 0 1 1 1
  line L145 (-66.9394, 36.306) -> (-66.9394, 34.9082)
  spline S291 degree 2 poles (-66.9394, 34.9082) (-66.9394, 34.5737) (-67.2923, 34.5737) knots 0 0 0 1 1 1
  spline S292 degree 2 poles (-67.2923, 34.5737) (-67.6498, 34.5737) (-67.6498, 34.9082) knots 0 0 0 1 1 1
  line L146 (-67.6498, 34.9082) -> (-67.6498, 36.306)
  spline S293 degree 2 poles (-68.7452, 36.306) (-68.7452, 36.6406) (-68.3968, 36.6406) knots 0 0 0 1 1 1
  spline S294 degree 2 poles (-68.3968, 36.6406) (-68.044, 36.6406) (-68.044, 36.306) knots 0 0 0 1 1 1
  line L147 (-68.044, 36.306) -> (-68.044, 34.9082)
  spline S295 degree 2 poles (-68.044, 34.9082) (-68.044, 34.5737) (-68.3968, 34.5737) knots 0 0 0 1 1 1
  spline S296 degree 2 poles (-68.3968, 34.5737) (-68.7452, 34.5737) (-68.7452, 34.9082) knots 0 0 0 1 1 1
  line L148 (-68.7452, 34.9082) -> (-68.7452, 36.306)
  spline S297 degree 2 poles (-14.9267, 49.0603) (-14.9267, 49.404) (-14.6289, 49.404) knots 0 0 0 1 1 1
  spline S298 degree 2 poles (-14.6289, 49.404) (-14.418, 49.404) (-14.253, 49.1703) knots 0 0 0 1 1 1
  line L149 (-14.253, 49.1703) -> (-11.187, 44.546)
  line L150 (-11.187, 44.546) -> (-11.187, 49.042)
  spline S299 degree 2 poles (-11.187, 49.042) (-11.187, 49.404) (-10.8295, 49.404) knots 0 0 0 1 1 1
  spline S300 degree 2 poles (-10.8295, 49.404) (-10.4766, 49.404) (-10.4766, 49.042) knots 0 0 0 1 1 1
  line L151 (-10.4766, 49.042) -> (-10.4766, 43.6386)
  spline S301 degree 2 poles (-10.4766, 43.6386) (-10.4766, 43.304) (-10.7974, 43.304) knots 0 0 0 1 1 1
  spline S302 degree 2 poles (-10.7974, 43.304) (-11.0266, 43.304) (-11.187, 43.5378) knots 0 0 0 1 1 1
  line L152 (-11.187, 43.5378) -> (-14.2255, 48.0841)
  line L153 (-14.2255, 48.0841) -> (-14.2255, 43.6661)
  spline S303 degree 2 poles (-14.2255, 43.6661) (-14.2255, 43.304) (-14.5784, 43.304) knots 0 0 0 1 1 1
  spline S304 degree 2 poles (-14.5784, 43.304) (-14.9267, 43.304) (-14.9267, 43.6661) knots 0 0 0 1 1 1
  line L154 (-14.9267, 43.6661) -> (-14.9267, 49.0603)
  spline S305 degree 2 poles (-20.2247, 48.9182) (-20.2476, 48.987) (-20.2476, 49.0511) knots 0 0 0 1 1 1
  spline S306 degree 2 poles (-20.2476, 49.0511) (-20.2476, 49.2024) (-20.0185, 49.3949) (-19.881, 49.3949) knots 0 0 0 1 2 2 2
  spline S307 degree 2 poles (-19.881, 49.3949) (-19.6473, 49.3949) (-19.5693, 49.1749) knots 0 0 0 1 1 1
  line L155 (-19.5693, 49.1749) -> (-19.2852, 48.4829)
  line L156 (-19.2852, 48.4829) -> (-17.0487, 48.4829)
  line L157 (-17.0487, 48.4829) -> (-16.7875, 49.1703)
  spline S308 degree 2 poles (-16.7875, 49.1703) (-16.6912, 49.3949) (-16.4575, 49.3949) knots 0 0 0 1 1 1
  spline S309 degree 2 poles (-16.4575, 49.3949) (-16.1046, 49.3949) (-16.1046, 49.0557) knots 0 0 0 1 1 1
  spline S310 degree 2 poles (-16.1046, 49.0557) (-16.1046, 48.9916) (-16.1229, 48.9366) knots 0 0 0 1 1 1
  line L158 (-16.1229, 48.9366) -> (-17.782, 44.5598)
  spline S311 degree 2 poles (-17.782, 44.5598) (-17.924, 44.3444) (-18.1349, 44.3444) knots 0 0 0 1 1 1
  spline S312 degree 2 poles (-18.1349, 44.3444) (-18.3457, 44.3444) (-18.4923, 44.5552) knots 0 0 0 1 1 1
  line L159 (-18.4923, 44.5552) -> (-20.2247, 48.9182)
  line L160 (-19.0515, 47.7862) -> (-18.144, 45.3985)
  line L161 (-18.144, 45.3985) -> (-17.2641, 47.7862)
  line L162 (-17.2641, 47.7862) -> (-19.0515, 47.7862)
  line L163 (-24.5282, 45.1143) -> (-23.3458, 45.1143)
  line L164 (-23.3458, 45.1143) -> (-23.3458, 49.042)
  spline S313 degree 2 poles (-23.3458, 49.042) (-23.3458, 49.4132) (-22.9883, 49.4132) knots 0 0 0 1 1 1
  spline S314 degree 2 poles (-22.9883, 49.4132) (-22.6262, 49.4132) (-22.6262, 49.042) knots 0 0 0 1 1 1
  line L165 (-22.6262, 49.042) -> (-22.6262, 45.1143)
  line L166 (-22.6262, 45.1143) -> (-21.4484, 45.1143)
  spline S315 degree 2 poles (-21.4484, 45.1143) (-21.0863, 45.1143) (-21.0863, 44.7523) knots 0 0 0 1 1 1
  spline S316 degree 2 poles (-21.0863, 44.7523) (-21.0863, 44.3902) (-21.4484, 44.3902) knots 0 0 0 1 1 1
  line L167 (-21.4484, 44.3902) -> (-24.5282, 44.3902)
  spline S317 degree 2 poles (-24.5282, 44.3902) (-24.8948, 44.3902) (-24.8948, 44.7523) knots 0 0 0 1 1 1
  spline S318 degree 2 poles (-24.8948, 44.7523) (-24.8948, 45.1143) (-24.5282, 45.1143) knots 0 0 0 1 1 1
  spline S319 degree 2 poles (-29.2212, 49.0328) (-29.2212, 49.3949) (-28.8729, 49.3949) knots 0 0 0 1 1 1
  spline S320 degree 2 poles (-28.8729, 49.3949) (-28.52, 49.3949) (-28.52, 49.0328) knots 0 0 0 1 1 1
  line L168 (-28.52, 49.0328) -> (-28.52, 47.0896)
  line L169 (-28.52, 47.0896) -> (-26.453, 47.0896)
  line L170 (-26.453, 47.0896) -> (-26.453, 49.0328)
  spline S321 degree 2 poles (-26.453, 49.0328) (-26.453, 49.3949) (-26.0956, 49.3949) knots 0 0 0 1 1 1
  spline S322 degree 2 poles (-26.0956, 49.3949) (-25.7427, 49.3949) (-25.7427, 49.0328) knots 0 0 0 1 1 1
  line L171 (-25.7427, 49.0328) -> (-25.7427, 44.7431)
  spline S323 degree 2 poles (-25.7427, 44.7431) (-25.7427, 44.3811) (-26.0956, 44.3811) knots 0 0 0 1 1 1
  spline S324 degree 2 poles (-26.0956, 44.3811) (-26.453, 44.3811) (-26.453, 44.7431) knots 0 0 0 1 1 1
  line L172 (-26.453, 44.7431) -> (-26.453, 46.3838)
  line L173 (-26.453, 46.3838) -> (-28.52, 46.3838)
  line L174 (-28.52, 46.3838) -> (-28.52, 44.7431)
  spline S325 degree 2 poles (-28.52, 44.7431) (-28.52, 44.3811) (-28.8729, 44.3811) knots 0 0 0 1 1 1
  spline S326 degree 2 poles (-28.8729, 44.3811) (-29.2212, 44.3811) (-29.2212, 44.7431) knots 0 0 0 1 1 1
  line L175 (-29.2212, 44.7431) -> (-29.2212, 49.0328)
  spline S327 degree 2 poles (-34.2992, 48.9182) (-34.3221, 48.987) (-34.3221, 49.0511) knots 0 0 0 1 1 1
  spline S328 degree 2 poles (-34.3221, 49.0511) (-34.3221, 49.2024) (-34.0929, 49.3949) (-33.9554, 49.3949) knots 0 0 0 1 2 2 2
  spline S329 degree 2 poles (-33.9554, 49.3949) (-33.7217, 49.3949) (-33.6438, 49.1749) knots 0 0 0 1 1 1
  line L176 (-33.6438, 49.1749) -> (-33.3597, 48.4829)
  line L177 (-33.3597, 48.4829) -> (-31.1231, 48.4829)
  line L178 (-31.1231, 48.4829) -> (-30.8619, 49.1703)
  spline S330 degree 2 poles (-30.8619, 49.1703) (-30.7657, 49.3949) (-30.5319, 49.3949) knots 0 0 0 1 1 1
  spline S331 degree 2 poles (-30.5319, 49.3949) (-30.179, 49.3949) (-30.179, 49.0557) knots 0 0 0 1 1 1
  spline S332 degree 2 poles (-30.179, 49.0557) (-30.179, 48.9916) (-30.1974, 48.9366) knots 0 0 0 1 1 1
  line L179 (-30.1974, 48.9366) -> (-31.8564, 44.5598)
  spline S333 degree 2 poles (-31.8564, 44.5598) (-31.9985, 44.3444) (-32.2093, 44.3444) knots 0 0 0 1 1 1
  spline S334 degree 2 poles (-32.2093, 44.3444) (-32.4201, 44.3444) (-32.5668, 44.5552) knots 0 0 0 1 1 1
  line L180 (-32.5668, 44.5552) -> (-34.2992, 48.9182)
  line L181 (-33.1259, 47.7862) -> (-32.2185, 45.3985)
  line L182 (-32.2185, 45.3985) -> (-31.3385, 47.7862)
  line L183 (-31.3385, 47.7862) -> (-33.1259, 47.7862)
  spline S335 degree 2 poles (-38.8409, 49.042) (-38.8409, 49.3949) (-38.5339, 49.3949) knots 0 0 0 1 1 1
  spline S336 degree 2 poles (-38.5339, 49.3949) (-38.3322, 49.3949) (-38.1993, 49.2024) knots 0 0 0 1 1 1
  line L184 (-38.1993, 49.2024) -> (-35.8528, 45.6093)
  line L185 (-35.8528, 45.6093) -> (-35.8528, 49.0328)
  spline S337 degree 2 poles (-35.8528, 49.0328) (-35.8528, 49.3949) (-35.5045, 49.3949) knots 0 0 0 1 1 1
  spline S338 degree 2 poles (-35.5045, 49.3949) (-35.1562, 49.3949) (-35.1562, 49.0328) knots 0 0 0 1 1 1